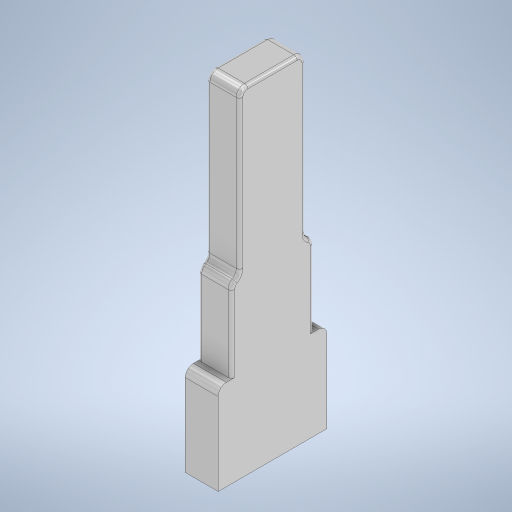
# Autodesk Inventor part: Slider
Saved by Autodesk Inventor 2023 (Build 270158000, 158)
## iProperties
Created: 2024-03-19
Part Number: Slider
Material: Generic
Document SubType Name: Modeling
Designer: noname
Density: 1 g/cm^3
Appearance: Aluminum - Polished
Author: noname
Autodesk Inventor part; units mm, degrees
ref_plane "YZ Plane" through (0, 0, 0) normal (1, 0, 0) x (0, 1, 0)
ref_plane "XZ Plane" through (0, 0, 0) normal (0, 1, 0) x (-1, 0, 0)
ref_plane "XY Plane" through (0, 0, 0) normal (0, 0, 1) x (1, 0, 0)
sketch "Sketch4" plane through (0, 0, 0) normal (1, 0, 0) x (0, 1, 0)
  line L0 (0, 0) -> (5.5, 0)
  line L1 (5.5, 0) -> (5.5, 6.6)
  line L2 (5.5, 6.6) -> (0, 6.6)
  line L3 (0, 6.6) -> (0, 0)
  line L4 (5.5, 5.8) -> (10.5, 5.8)
  line L5 (10.5, 5.8) -> (10.5, 0.8)
  line L6 (10.5, 0.8) -> (5.5, 0.8)
  line L7 (5.5, 0.8) -> (5.5, 5.8)
  line L8 (0, 3.3) -> (20.5, 3.3)
  line L9 (10.5, 5.3) -> (20.5, 5.3)
  line L10 (20.5, 5.3) -> (20.5, 1.3)
  line L11 (20.5, 1.3) -> (10.5, 1.3)
  line L12 (10.5, 1.3) -> (10.5, 5.3)
  dimension "d0" = 6.6
  dimension "d1" = 5.5
  dimension "d2" = 5
  dimension "d3" = 4
  dimension "d4" = 15
  dimension "d5" = 10
  constraints: 26 end point, 6 parallel, 4 horizontal, 3 perpendicular, 2 midpoint, 2 point on line, 1 other
  measures "d0" distance between parallel lines of L0 L2
  measures "d1" distance between parallel lines of L3 L1
  measures "d2" distance between parallel lines of L6 L4
  measures "d3" distance between parallel lines of L11 L9
  measures "d4" distance between parallel lines of L1 L10
  measures "d5" distance between parallel lines of L10 L5
extrude "Extrusion1" add sketch "Sketch4" along normal blind 2
fillet "Fillet1" radius 0.5 8 edges at (1, 10.5, 5.3) (1, 20.5, 5.3) (1, 10.5, 5.8) (1, 20.5, 1.3) (1, 10.5, 1.3) (1, 10.5, 0.8) (1, 5.5, 0) (1, 5.5, 6.6)
fillet "Fillet2" radius 0.2 18 edges at (2, 10.3837, 5.7329) (2, 15.4995, 5.3) (2, 20.3536, 5.1536) (2, 20.5, 3.3) (2, 20.3536, 1.4464) (2, 15.4995, 1.3) (2, 10.3837, 0.8671) (2, 7.8168, 0.8) (2, 7.8168, 5.8) (0, 10.3837, 5.7329) (0, 15.4995, 5.3) (0, 20.3536, 5.1536) (0, 20.5, 3.3) (0, 20.3536, 1.4464) (0, 15.4995, 1.3) (0, 10.3837, 0.8671) (0, 7.8168, 0.8) (0, 7.8168, 5.8)
body "Solid1"
